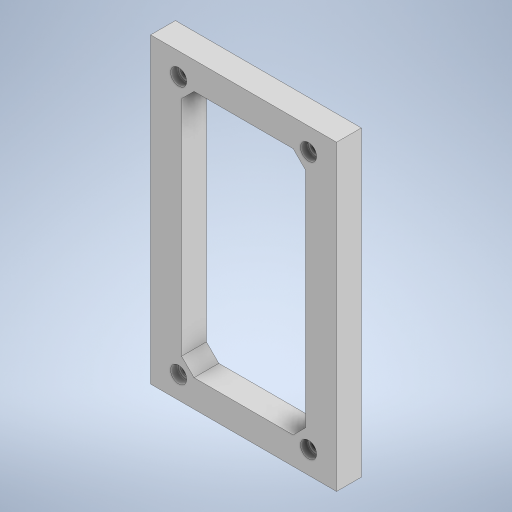
# Autodesk Inventor part: 조면 스위치 단차
Saved by Autodesk Inventor 2023 (Build 270158000, 158)
## iProperties
Created: 2022-09-06
Part Number: 조면 스위치 단차
Material: 일반
Document SubType Name: Modeling
Designer: user
Density: 1 g/cm^3
Appearance: 기본값
Author: user
Autodesk Inventor part; units mm, degrees
ref_plane "YZ Plane" through (0, 0, 0) normal (1, 0, 0) x (0, 1, 0)
ref_plane "XZ Plane" through (0, 0, 0) normal (0, 1, 0) x (-1, 0, 0)
ref_plane "XY Plane" through (0, 0, 0) normal (0, 0, 1) x (1, 0, 0)
sketch "스케치1" plane through (0, 0, 0) normal (0, 0, 1) x (1, 0, 0)
  line L0 (-26.2, -52) -> (26.2, -52) construction
  line L1 (26.2, -52) -> (26.2, 52) construction
  line L2 (26.2, 52) -> (-26.2, 52) construction
  line L3 (-26.2, 52) -> (-26.2, -52) construction
  line L4 (-26.2, -52) -> (26.2, 52) construction
  line L5 (26.2, -52) -> (-26.2, 52) construction
  circle A0 centre (-26.2, 52) radius 2.25
  line L6 (0, 0) -> (0, 20.7433)
  line L7 (0, 0) -> (13.3788, 0)
  circle A1 centre (26.2, 52) radius 2.25
  line L8 (26.2, -52) -> (-26.2, -52) construction
  circle A2 centre (-26.2, -52) radius 2.25
  circle A3 centre (26.2, -52) radius 2.25
  line L9 (-37.5, -61) -> (37.5, -61)
  line L10 (37.5, -61) -> (37.5, 61)
  line L11 (37.5, 61) -> (-37.5, 61)
  line L12 (-37.5, 61) -> (-37.5, -61)
  line L13 (-37.5, -61) -> (37.5, 61) construction
  line L14 (37.5, -61) -> (-37.5, 61) construction
  line L15 (20, -50) -> (-20, -50)
  line L16 (-25, -45) -> (-25, 45)
  line L17 (-20, 50) -> (20, 50)
  line L18 (25, 45) -> (25, -45)
  line L19 (25, -50) -> (-25, 50) construction
  line L20 (-25, -50) -> (25, 50) construction
  line L21 (-25, 45) -> (-20, 50)
  line L22 (20, 50) -> (25, 45)
  line L23 (25, -45) -> (20, -50)
  line L24 (-20, -50) -> (-25, -45)
  dimension "d0" = 52.4
  dimension "d1" = 104
  dimension "d2" = 4.5
  dimension "d3" = 75
  dimension "d4" = 122
  dimension "d5" = 50
  dimension "d6" = 100
  dimension "d7" = 5
  dimension "d8" = 5
  dimension "d9" = 5
  dimension "d10" = 5
  dimension "d11" = 5
  dimension "d12" = 5
  dimension "d13" = 5
  dimension "d14" = 5
  constraints: 50 end point, 8 point on line, 6 midpoint, 6 parallel, 4 centre point, 4 coincident, 4 horizontal, 3 perpendicular, 3 symmetric about line, 1 vertical, 3 other
  measures "d0" distance of L1.end L2.end
  measures "d1" distance of L0.end L1.end
  measures "d2" diameter of A0
  measures "d3" distance of L11.end L10.end
  measures "d4" distance of L10.end L9.end
  measures "d5" distance of L19.end L20.end
  measures "d6" distance of L20.start L19.end
  measures "d7" distance of L16.end L19.end
  measures "d8" distance of L17.start L19.end
  measures "d9" distance of L17.end L20.end
  measures "d10" distance of L18.start L20.end
  measures "d11" distance of L18.end L19.start
  measures "d12" distance of L15.start L19.start
  measures "d13" distance of L15.end L20.start
  measures "d14" distance of L16.start L20.start
extrude "돌출1" add sketch "스케치1" along normal blind 10
sketch "스케치2" plane through (0, 0, 10) normal (0, 0, 1) x (1, 0, 0)
  circle A0 centre (-26.2, 52) radius 2.25 projected
  circle A1 centre (-26.2, 52) radius 3.25
  circle A2 centre (26.2, 52) radius 2.25 projected
  circle A3 centre (26.2, 52) radius 3.25
  circle A4 centre (-26.2, -52) radius 2.25 projected
  circle A5 centre (-26.2, -52) radius 3.25
  circle A6 centre (26.2, -52) radius 2.25 projected
  circle A7 centre (26.2, -52) radius 3.25
  point P0 (0, 0)
  dimension "d17" = 6.5
  dimension "d18" = 6.5
  dimension "d19" = 6.5
  dimension "d20" = 6.5
  constraints: 4 centre point, 4 coincident
  measures "d17" diameter of A1
  measures "d18" diameter of A3
  measures "d19" diameter of A5
  measures "d20" diameter of A7
extrude "돌출2" cut sketch "스케치2" against normal blind 3 contours A0 | A1 | A2 | A3 | A4 | A5 | A6 | A7
equation "\"d8\" = d7"
equation "\"d9\" = d7"
equation "\"d10\" = d9"
equation "\"d11\" = d7"
equation "\"d12\" = d11"
equation "\"d13\" = d7"
equation "\"d14\" = d13"
